Autodesk Inventor part; units mm, degrees
(part 2 of 2)
sketch "Sketch20" plane through (0, 82.55, 0) normal (0, -1, 0) x (1, 0, 0)
  circle A0 centre (19.4937, -17.0126) radius 2.05 projected
  circle A1 centre (19.4937, -56.0126) radius 2.05 projected
  circle A2 centre (-19.5063, -17.0126) radius 2.05 projected
  circle A3 centre (-19.5063, -56.0126) radius 2.05 projected
  line L0 (-47.625, -81.28) -> (-47.625, -60.7421) projected
  arc A4 (-47.625, -81.28) -> (-46.355, -82.55) centre (-46.355, -81.28) ccw projected
  line L1 (-25.8171, -82.55) -> (-46.355, -82.55) projected
  line L2 (-23.2771, -80.01) -> (-25.8171, -82.55) projected
  line L3 (23.2771, -80.01) -> (-23.2771, -80.01) projected
  line L4 (25.8171, -82.55) -> (23.2771, -80.01) projected
  line L5 (46.355, -82.55) -> (25.8171, -82.55) projected
  arc A5 (46.355, -82.55) -> (47.625, -81.28) centre (46.355, -81.28) ccw projected
  line L6 (47.625, -60.7421) -> (47.625, -81.28) projected
  line L7 (45.085, -58.2021) -> (47.625, -60.7421) projected
  line L8 (45.085, 58.2021) -> (45.085, -58.2021) projected
  line L9 (47.625, 60.7421) -> (45.085, 58.2021) projected
  line L10 (47.625, 81.28) -> (47.625, 60.7421) projected
  arc A6 (47.625, 81.28) -> (46.355, 82.55) centre (46.355, 81.28) ccw projected
  line L11 (25.8171, 82.55) -> (46.355, 82.55) projected
  line L12 (23.2771, 80.01) -> (25.8171, 82.55) projected
  line L13 (-23.2771, 80.01) -> (23.2771, 80.01) projected
  line L14 (-25.8171, 82.55) -> (-23.2771, 80.01) projected
  line L15 (-46.355, 82.55) -> (-25.8171, 82.55) projected
  arc A7 (-46.355, 82.55) -> (-47.625, 81.28) centre (-46.355, 81.28) ccw projected
  line L16 (-47.625, 60.7421) -> (-47.625, 81.28) projected
  line L17 (-45.085, 58.2021) -> (-47.625, 60.7421) projected
  line L18 (-45.085, -58.2021) -> (-45.085, 58.2021) projected
  line L19 (-47.625, -60.7421) -> (-45.085, -58.2021) projected
  point P0 (0, 0)
  dimension "d0" = 82.55
  dimension "d1" = 152.4
  dimension "d2" = 3.81
  dimension "d3" = 2.54
  dimension "d4" = 2.54
  dimension "d5" = 25.4
  dimension "d6" = 25.4
  dimension "d7" = 2.54
  dimension "d8" = 2.54
  dimension "d9" = 2.54
  dimension "d10" = 2.54
chamfer "Chamfer3" distance 0.5 angle 45 34 edges at (-24.9559, 85.725, 33.5842) (-19.4994, 85.725, 29.0887) (-28.7866, 85.725, 37.178) (-24.9839, 85.725, 40.7415) (-19.5975, 85.725, 45.3352) (-20.1621, 85.725, 52.3858) (-15.1905, 85.725, 57.5187) (-20.2937, 85.725, 57.5893) (-7.0569, 85.725, 51.5657) (-10.3182, 85.725, 56.3273) (-11.7525, 85.725, 55.5867) (-0.0042, 85.725, 27.0641) (7.0484, 85.09, 51.5657) (10.3097, 85.725, 56.3273) (11.744, 85.725, 55.5867) (15.1821, 85.725, 57.5187) (20.2853, 85.725, 57.5893) (20.1536, 85.725, 52.3858) (19.5891, 85.725, 45.3352) (24.9754, 85.725, 40.7415) (28.7782, 85.725, 37.178) (24.9475, 85.725, 33.5842) (19.4909, 85.725, 29.0887) (20.1177, 85.725, 22.0371) (20.325, 85.725, 16.7283) (14.9665, 85.725, 16.9612) (8.1463, 85.725, 17.7431) (3.8488, 85.725, 12.2699) (-0.0042, 85.725, 8.2665) (-3.8573, 85.725, 12.2699) (-8.1548, 85.725, 17.7431) (-14.975, 85.725, 16.9612) (-20.3335, 85.725, 16.7283) (-20.1262, 85.725, 22.0371)
chamfer "Chamfer4" distance 0.5 angle 45 35 edges at (21.3733, 85.09, 58.6782) (15.2226, 85.09, 59.4119) (10.1957, 85.09, 58.1186) (5.6844, 85.09, 51.9961) (7.7711, 85.09, 57.3965) (8.128, 85.09, 58.3202) (3.3984, 85.09, 46.0799) (22.014, 85.09, 52.3846) (21.0114, 85.09, 45.9237) (26.2991, 85.09, 42.062) (30.3174, 85.09, 37.1821) (26.262, 85.09, 32.2687) (20.9107, 85.09, 28.4939) (21.9911, 85.09, 22.0257) (21.4139, 85.09, 15.6403) (14.9696, 85.09, 15.0979) (8.7345, 85.09, 16.3206) (5.157, 85.09, 10.9489) (-0.0042, 85.09, 6.7273) (-5.1655, 85.09, 10.9489) (-8.743, 85.09, 16.3206) (-14.9781, 85.09, 15.0979) (-21.4224, 85.09, 15.6403) (-21.9996, 85.09, 22.0257) (-20.9192, 85.09, 28.4939) (-26.2704, 85.09, 32.2687) (-30.3259, 85.09, 37.1821) (-26.3076, 85.09, 42.062) (-21.0199, 85.09, 45.9237) (-22.0224, 85.09, 52.3846) (-21.3817, 85.09, 58.6782) (-15.231, 85.09, 59.4119) (-10.2042, 85.09, 58.1186) (-5.7726, 85.09, 52.2023) (-0.0042, 85.09, 28.6025)
chamfer "Chamfer5" [suppressed]
sketch "Sketch21" plane through (43.715, 24.13, 78.64) normal (0, 0, -1) x (-1, 0, 0)
  line L0 (0, 0) -> (0, 58.42) projected
  line L1 (87.43, 0) -> (0, 0) projected
  line L2 (87.43, 0) -> (87.43, 58.42) projected
  line L3 (0, 58.42) -> (87.43, 58.42) projected
  line L4 (0, 58.42) -> (87.43, 58.42)
  line L5 (87.43, 58.42) -> (87.43, 55.88)
  line L6 (87.43, 55.88) -> (0, 55.88)
  line L7 (0, 55.88) -> (0, 58.42)
  point P0 (43.715, -24.13)
  dimension "d158" = 2.54
  constraints: 8 end point, 2 parallel, 1 horizontal, 1 perpendicular, 1 point on line
  measures "d158" distance of L4.end L5.end
extrude "Extrusion21" add sketch "Sketch21" along normal up to surface (157.28 mm away) contours L0 L3 L2 L6 bodies 2
extrude "Extrusion22" [suppressed]
sketch "Sketch24" plane through (-43.715, 80.01, 78.64) normal (0, -1, 0) x (1, 0, 0)
  circle A0 centre (43.7087, -115.1526) radius 11.303 projected
  circle A1 centre (43.7087, -115.1526) radius 24.003 projected
  circle A2 centre (43.7087, -115.1526) radius 18.923 projected
  circle A3 centre (43.7087, -115.1526) radius 17.653 projected
  circle A4 centre (43.7087, -115.1526) radius 12.573 projected
  line L0 (55.9865, -100.7534) -> (59.5875, -97.1524) projected
  line L1 (55.0855, -101.6545) -> (51.475, -105.2649) projected
  line L2 (46.9186, -109.8213) -> (50.5698, -106.1702) projected
  circle A5 centre (43.7087, -115.1526) radius 6.223 projected
  line L3 (34.7263, -122.0136) -> (38.3775, -118.3625) projected
  line L4 (30.2106, -126.5293) -> (33.8211, -122.9188) projected
  line L5 (29.3096, -127.4304) -> (25.7085, -131.0314) projected
  line L6 (38.3775, -111.9426) -> (34.7263, -108.2915) projected
  line L7 (40.4988, -109.8213) -> (36.8476, -106.1702) projected
  line L8 (32.3319, -101.6545) -> (35.9424, -105.2649) projected
  line L9 (30.2106, -103.7758) -> (33.8211, -107.3863) projected
  line L10 (29.3096, -102.8747) -> (25.7085, -99.2737) projected
  line L11 (31.4309, -100.7534) -> (27.8299, -97.1524) projected
  line L12 (58.1078, -102.8747) -> (61.7089, -99.2737) projected
  line L13 (57.2068, -103.7758) -> (53.5963, -107.3863) projected
  line L14 (49.0399, -111.9426) -> (52.6911, -108.2915) projected
  line L15 (52.6911, -122.0136) -> (49.0399, -118.3625) projected
  line L16 (50.5698, -124.1349) -> (46.9186, -120.4838) projected
  line L17 (55.0855, -128.6506) -> (51.475, -125.0402) projected
  line L18 (57.2068, -126.5293) -> (53.5963, -122.9188) projected
  line L19 (55.9865, -129.5517) -> (59.5875, -133.1527) projected
  line L20 (58.1078, -127.4304) -> (61.7089, -131.0314) projected
  line L21 (32.3319, -128.6506) -> (35.9424, -125.0402) projected
  line L22 (36.8476, -124.1349) -> (40.4988, -120.4838) projected
  line L23 (31.4309, -129.5517) -> (27.8299, -133.1527) projected
  circle A6 centre (63.2087, -95.6526) radius 2.05 projected
  circle A7 centre (24.2087, -95.6526) radius 2.05 projected
  circle A8 centre (24.2087, -134.6526) radius 2.05 projected
  circle A9 centre (63.2087, -134.6526) radius 2.05 projected
  point P0 (43.715, -78.64)
  constraints: 6 other
extrude "Extrusion24" cut sketch "Sketch18" along normal mid plane 25.4 contours A13 L44 A12 L16 | L30 A12 L54 A13 | A13 L26 A12 L61 | A11 L46 A10 L18 | L63 A12 L40 A13 | L32 A10 L52 A11 | A11 L24 A10 L58 | A9 L48 A8 L20 | L65 A10 L38 A11 | L34 A8 L50 A9 | A9 L22 A8 L57 | L67 A8 L36 A9 bodies 3
extrude "Extrusion25" cut sketch "Sketch18" along normal mid plane 50.8 contours L15 A7 L29 | A7 L15 | L29 A7 | L43 A4 | A4 L62 L43 | L16 A12 L30 A13 | A13 L44 A12 L16 | A4 L62 | L30 A12 L54 A13 | A13 L61 A12 L44 | L17 A11 L31 A12 | A12 L45 A11 L17 | L55 A5 L68 | A5 L55 | L54 A12 L63 A13 | L31 A11 L53 A12 | A13 L26 A12 L61 | A12 L60 A11 L45 | L18 A10 L32 A11 | A11 L46 A10 L18 | L68 A5 | L63 A12 L40 A13 | L53 A11 L64 A12 | L32 A10 L52 A11 | A12 L25 A11 L60 | A11 L58 A10 L46 | L19 A9 L33 A10 | A10 L47 A9 L19 | L27 A6 | A6 L41 L27 | L40 A12 L26 A13 | L64 A11 L39 A12 | L52 A10 L65 A11 | L33 A9 L51 A10 | A11 L24 A10 L58 | A10 L59 A9 L47 | L20 A8 L34 A9 | A9 L48 A8 L20 | A6 L41 | L39 A11 L25 A12 | L65 A10 L38 A11 | L51 A9 L66 A10 | L34 A8 L50 A9 | A10 L23 A9 L59 | A9 L57 A8 L48 | L21 L49 L35 A8 | A8 L49 L21 | L38 A10 L24 A11 | L66 A9 L37 A10 | L50 A8 L67 A9 | L35 L49 A8 | A9 L22 A8 L57 | A8 L56 L21 L49 | L21 L56 L35 L49 | L37 A9 L23 A10 | L67 A8 L36 A9 | L49 L35 L56 A8 | A8 L21 L56 | L21 A8 L35 L56 | L36 A8 L22 A9 | L56 L35 A8 bodies 2
fillet "Fillet7" radius 1.27 48 edges at (5.3249, 84.1375, -39.7225) (-3.2162, 84.1375, -31.1813) (-7.7726, 84.1375, -26.6249) (-12.2841, 84.1375, -22.1134) (-11.3831, 84.1375, -23.0145) (-15.8851, 84.1375, -18.5124) (-6.8674, 84.1375, -27.5302) (3.2036, 84.1375, -31.1813) (6.8548, 84.1375, -27.5302) (7.76, 84.1375, -26.6249) (11.3705, 84.1375, -23.0145) (12.2715, 84.1375, -22.1134) (15.8725, 84.1375, -18.5124) (17.9939, 84.1375, -20.6337) (14.3928, 84.1375, -24.2347) (13.4918, 84.1375, -25.1358) (9.8813, 84.1375, -28.7463) (8.9761, 84.1375, -29.6515) (5.3249, 84.1375, -33.3026) (8.9761, 84.1375, -43.3736) (9.8813, 84.1375, -44.2788) (13.4918, 84.1375, -47.8893) (14.3928, 84.1375, -48.7904) (17.9939, 84.1375, -52.3914) (-5.3375, 84.1375, -33.3026) (-8.9887, 84.1375, -29.6515) (-9.8939, 84.1375, -28.7463) (-13.5044, 84.1375, -25.1358) (-14.4054, 84.1375, -24.2347) (-18.0065, 84.1375, -20.6337) (-5.3375, 84.1375, -39.7225) (-8.9887, 84.1375, -43.3736) (-9.8939, 84.1375, -44.2788) (-13.5044, 84.1375, -47.8893) (-14.4054, 84.1375, -48.7904) (-18.0065, 84.1375, -52.3914) (-15.8851, 84.1375, -54.5127) (-12.2841, 84.1375, -50.9117) (-11.3831, 84.1375, -50.0106) (-7.7726, 84.1375, -46.4002) (-6.8674, 84.1375, -45.4949) (-3.2162, 84.1375, -41.8438) (3.2036, 84.1375, -41.8438) (6.8548, 84.1375, -45.4949) (7.76, 84.1375, -46.4002) (11.3705, 84.1375, -50.0106) (12.2715, 84.1375, -50.9117) (15.8725, 84.1375, -54.5127)
sketch "Sketch25" plane through (-43.715, 80.01, 78.64) normal (0, -1, 0) x (1, 0, 0)
  line L0 (85.2202, -2.2098) -> (2.2202, -2.2098)
  line L1 (2.2202, -2.2098) -> (2.2202, -70.2098)
  line L2 (2.2202, -70.2098) -> (85.2202, -70.2098)
  line L3 (85.2202, -70.2098) -> (85.2202, -2.2098)
  circle A0 centre (63.2087, -134.6526) radius 2.05 projected
  circle A1 centre (63.2087, -95.6526) radius 2.05 projected
  circle A2 centre (24.2087, -134.6526) radius 2.05 projected
  circle A3 centre (43.7087, -115.1526) radius 24.003 projected
  circle A4 centre (24.2087, -95.6526) radius 2.05 projected
  line L4 (87.43, -157.28) -> (0, -157.28) projected
  line L5 (87.43, 0) -> (87.43, -157.28) projected
  line L6 (0, 0) -> (87.43, 0) projected
  line L7 (0, -157.28) -> (0, 0) projected
  line L8 (85.2202, -2.2098) -> (80.1402, -2.2098)
  line L9 (80.1402, -2.2098) -> (80.1402, -7.2898)
  line L10 (80.1402, -7.2898) -> (85.2202, -7.2898)
  line L11 (85.2202, -7.2898) -> (85.2202, -2.2098)
  circle A5 centre (80.1402, -7.2898) radius 1.7526
  circle A6 centre (80.1402, -7.2898) radius 3.0226
  line L12 (85.2202, -36.2098) -> (82.6802, -36.2098)
  line L13 (43.7202, -2.2098) -> (43.7202, -3.0754)
  circle A7 centre (80.1402, -7.2898) radius 5.5626
  circle A8 centre (80.1402, -65.1298) radius 1.7526
  circle A9 centre (80.1402, -65.1298) radius 3.0226
  circle A10 centre (80.1402, -65.1298) radius 5.5626
  circle A11 centre (7.3002, -7.2898) radius 1.7526
  circle A12 centre (7.3002, -7.2898) radius 3.0226
  circle A13 centre (7.3002, -7.2898) radius 5.5626
  circle A14 centre (7.3002, -65.1298) radius 5.5626
  circle A15 centre (7.3002, -65.1298) radius 3.0226
  circle A16 centre (7.3002, -65.1298) radius 1.7526
  point P0 (43.715, -78.64)
  dimension "d174" = 83
  dimension "d175" = 68
  dimension "d176" = 2.2098
  dimension "d177" = 2.2098
  dimension "d178" = 5.08
  dimension "d179" = 5.08
  dimension "d180" = 3.5052
  dimension "d181" = 1.27
  dimension "d182" = 2.54
  constraints: 20 end point, 12 centre point, 4 parallel, 3 horizontal, 3 symmetric about line, 2 midpoint, 2 perpendicular, 1 coincident, 1 vertical, 9 other
  measures "d174" distance of L2.end L1.end
  measures "d175" distance of L1.end L0.end
  measures "d176" distance between parallel lines of L5 L3
  measures "d177" distance between parallel lines of L6 L0
  measures "d178" distance of L10.end L9.end
  measures "d179" distance of L9.end L8.end
  measures "d180" diameter of A5
  measures "d181" radial gap between concentric circles of A5 A6
  measures "d182" radial gap between concentric circles of A6 A7
ref_plane "Work Plane3" through (-36.4148, 67.31, 71.3502) normal (0, -1, 0) x (1, 0, 0)
extrude "Extrusion27" add sketch "Sketch25" along normal up to surface (12.7 mm away) contours A7 L3 L10 A6 L9 L0 | L0 A7 | A7 L3 | L9 A6 L10 L3 A7 L0 | A6 L10 A5 L9 | L9 A5 L10 A6 | A13 L1 L0 | L0 A13 | A10 L3 | L3 A10 L2 | L1 A13 | L2 A10 | A14 L2 L1 | L1 A14 | A14 L2 | A9 | A12 | A15 picked at (7.4216, -2.9029) picked at (80.2616, -69.5167) picked at (7.4216, -69.5167) bodies 2
chamfer "Chamfer6" distance 2.54 angle 75 1 edges at (-41.9774, 67.31, 71.3502) measured on face at (-41.4774, 67.31, 71.3502)
chamfer "Chamfer7" distance 2.54 angle 75 1 edges at (30.8626, 67.31, 71.3502) measured on face at (31.3626, 67.31, 71.3502)
chamfer "Chamfer8" distance 2.54 angle 75 1 edges at (-41.9774, 67.31, 13.5102) measured on face at (-41.4774, 67.31, 13.5102)
chamfer "Chamfer9" distance 2.54 angle 75 1 edges at (30.8626, 67.31, 13.5102) measured on face at (31.3626, 67.31, 13.5102)
chamfer "Chamfer10" distance 1.27 angle 45 4 edges at (17.4437, 85.725, -17.0126) (17.4437, 85.725, -56.0126) (-21.5563, 85.725, -56.0126) (-21.5563, 85.725, -17.0126)
chamfer "Chamfer11" distance 0.254 angle 45 96 edges at (-24.0093, 85.725, -36.5126) (-17.9974, 85.725, -51.7764) (-16.1162, 85.725, -50.5011) (-14.8416, 85.725, -48.7848) (-18.9293, 85.725, -36.5126) (-14.8416, 85.725, -24.2403) (-16.1162, 85.725, -22.524) (-17.9974, 85.725, -21.2487) (-0.0063, 85.725, -60.5156) (15.2575, 85.725, -54.5036) (13.9823, 85.725, -52.6225) (12.266, 85.725, -51.3479) (-0.0063, 85.725, -55.4356) (-12.2786, 85.725, -51.3479) (-13.9949, 85.725, -52.6225) (-15.2701, 85.725, -54.5036) (-0.0063, 85.725, -54.1656) (10.7182, 85.725, -49.9967) (9.4372, 85.725, -48.0773) (7.7532, 85.725, -46.7982) (-0.0063, 85.725, -49.0856) (-7.7658, 85.725, -46.7982) (-9.4498, 85.725, -48.0773) (-10.7308, 85.725, -49.9967) (-17.6593, 85.725, -36.5126) (-13.4905, 85.725, -47.237) (-11.5711, 85.725, -45.956) (-10.2919, 85.725, -44.2721) (-12.5793, 85.725, -36.5126) (-10.2919, 85.725, -28.753) (-11.5711, 85.725, -27.0691) (-13.4905, 85.725, -25.7881) (-11.3093, 85.725, -36.5126) (-8.9607, 85.725, -42.6301) (-6.9378, 85.725, -41.3227) (-5.6407, 85.725, -39.7159) (-6.2293, 85.725, -36.5126) (-5.6407, 85.725, -33.3092) (-6.9378, 85.725, -31.7024) (-8.9607, 85.725, -30.395) (-0.0063, 85.725, -47.8156) (6.1113, 85.725, -45.4669) (4.8039, 85.725, -43.444) (3.197, 85.725, -42.1469) (-0.0063, 85.725, -42.7356) (-3.2096, 85.725, -42.1469) (-4.8165, 85.725, -43.444) (-6.1239, 85.725, -45.4669) (6.9252, 85.725, -41.3227) (8.9481, 85.725, -42.6301) (11.2967, 85.725, -36.5126) (8.9481, 85.725, -30.395) (6.9252, 85.725, -31.7024) (5.6281, 85.725, -33.3092) (6.2167, 85.725, -36.5126) (5.6281, 85.725, -39.7159) (-0.0063, 85.725, -30.2896) (3.197, 85.725, -30.8782) (4.8039, 85.725, -29.5811) (6.1113, 85.725, -27.5582) (-0.0063, 85.725, -25.2096) (-6.1239, 85.725, -27.5582) (-4.8165, 85.725, -29.5811) (-3.2096, 85.725, -30.8782) (-0.0063, 85.725, -23.9396) (7.7532, 85.725, -26.2269) (9.4372, 85.725, -24.9478) (10.7182, 85.725, -23.0284) (-0.0063, 85.725, -18.8596) (-10.7308, 85.725, -23.0284) (-9.4498, 85.725, -24.9478) (-7.7658, 85.725, -26.2269) (12.5667, 85.725, -36.5126) (10.2793, 85.725, -44.2721) (11.5585, 85.725, -45.956) (13.4779, 85.725, -47.237) (17.6467, 85.725, -36.5126) (13.4779, 85.725, -25.7881) (11.5585, 85.725, -27.0691) (10.2793, 85.725, -28.753) (18.9167, 85.725, -36.5126) (14.829, 85.725, -48.7848) (16.1036, 85.725, -50.5011) (17.9848, 85.725, -51.7764) (23.9967, 85.725, -36.5126) (17.9848, 85.725, -21.2487) (16.1036, 85.725, -22.524) (14.829, 85.725, -24.2403) (-0.0063, 85.725, -17.5896) (12.266, 85.725, -21.6772) (13.9823, 85.725, -20.4026) (15.2575, 85.725, -18.5215) (-0.0063, 85.725, -12.5096) (-15.2701, 85.725, -18.5215) (-13.9949, 85.725, -20.4026) (-12.2786, 85.725, -21.6772)
sketch "Sketch28" plane through (47.625, 31.75, 57.15) normal (1, 0, 0) x (0, 0, -1)
  line L0 (114.3, -34.29) -> (114.3, 0) projected
  line L1 (0, 0) -> (114.3, 0) projected
  line L2 (0, -34.29) -> (0, 0) projected
  line L3 (114.3, -34.29) -> (0, -34.29) projected
  line L4 (0, 0) -> (5.08, 0)
  line L5 (5.08, 0) -> (5.08, -3.81)
  line L6 (5.08, -3.81) -> (0, -3.81)
  line L7 (0, -3.81) -> (0, 0)
  circle A0 centre (5.08, -3.81) radius 0.9
  line L8 (57.15, 0) -> (57.15, -1.0158)
  circle A1 centre (109.22, -3.81) radius 0.9
  point P0 (57.15, -31.75)
  dimension "d208" = 5.08
  dimension "d209" = 3.81
  dimension "d210" = 1.8
  constraints: 10 end point, 2 centre point, 2 parallel, 1 coincident, 1 horizontal, 1 midpoint, 1 perpendicular, 1 symmetric about line, 1 vertical, 1 other
  measures "d208" distance of L5.end L6.end
  measures "d209" distance of L4.end L5.end
  measures "d210" diameter of A0
ref_plane "Work Plane4" through (47.625, 31.75, 57.15) normal (1, 0, 0) x (0, 0, -1)
sketch "Sketch29" plane through (47.625, 31.75, 57.15) normal (1, 0, 0) x (0, 0, -1)
  circle A0 centre (5.08, -3.81) radius 0.9 projected
  circle A1 centre (109.22, -3.81) radius 0.9 projected
  point P0 (57.15, -31.75)
extrude "Extrusion29" cut sketch "Sketch29" against normal through all bodies 1
extrude "Extrusion30" cut sketch "Sketch28" against normal through all contours A0 L5 L6 | L6 L5 A0 | A1 bodies 2
sketch "Sketch30" plane through (0, 85.09, 0) normal (0, 1, 0) x (1, 0, 0)
  line L0 (-47.625, -82.55) -> (-38.735, -82.55)
  line L1 (-38.735, -82.55) -> (-38.735, -73.66)
  line L2 (-38.735, -73.66) -> (-47.625, -73.66)
  line L3 (-47.625, -73.66) -> (-47.625, -82.55)
  circle A0 centre (-38.735, -73.66) radius 1.7526
  point P0 (0, 0)
  dimension "d217" = 8.89
  dimension "d218" = 8.89
  dimension "d219" = 3.5052
  constraints: 8 end point, 2 parallel, 1 centre point, 1 coincident, 1 horizontal, 1 perpendicular
  measures "d217" distance of L2.end L1.end
  measures "d218" distance of L1.end L0.end
  measures "d219" diameter of A0
equation "\"d80\" = d79"
equation "\"d81\" = d79"
equation "\"d82\" = d81"
equation "\"d83\" = d79"
equation "\"d84\" = d83"
equation "\"d85\" = d79"
equation "\"d86\" = d85"
body "Solid1"
body "Solid2"
body "Solid4"
